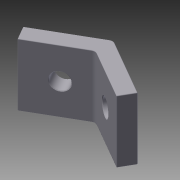
# Autodesk Inventor part: drive_frame_bracket
Saved by Autodesk Inventor 2012 (Build 160160000, 160)
## iProperties
Created: 2012-10-26
Part Number: drive_frame_bracket
Material: Aluminum-6061
Document SubType Name: Modeling
Designer: agmlego
Mass: 115.378 g
Surface Area: 72.2331 cm^2
Volume: 42.5748 cm^3
Density: 2.71 g/cm^3
Author: agmlego
Autodesk Inventor part; units mm, degrees
ref_plane "YZ Plane" through (0, 0, 0) normal (1, 0, 0) x (0, 1, 0)
ref_plane "XZ Plane" through (0, 0, 0) normal (0, 1, 0) x (-1, 0, 0)
ref_plane "XY Plane" through (0, 0, 0) normal (0, 0, 1) x (1, 0, 0)
sketch "Sketch1" plane through (0, 0, 0) normal (0, 0, 1) x (1, 0, 0)
  line L0 (-0.0175, -6.5307) -> (-20.2143, -18.1913)
  line L1 (-23.3893, -12.6921) -> (-0.0175, 0.8017)
  line L2 (-0.0175, 0.8017) -> (23.3544, -12.6921)
  line L3 (20.1794, -18.1913) -> (-0.0175, -6.5307)
  line L4 (-0.0175, 0.8017) -> (-0.0175, -6.5307) construction
  line L5 (-20.2143, -18.1913) -> (-23.3893, -12.6921)
  line L6 (20.1794, -18.1913) -> (23.3544, -12.6921)
  dimension "d4" = 120
  dimension "d5" = 6.35
  dimension "d6" = 26.9875
  constraints: 14 end point, 2 equal length, 2 parallel, 2 perpendicular
  measures "d4" angle of L2 L1
  measures "d5" distance between parallel lines of L0 L1
  measures "d6" distance from line of L1.end L5
extrude "Extrusion1" add sketch "Sketch1" along normal blind 25.4
hole "Hole1" at (9.1809, -11.8413, 12.7) direction (0.5, 0.8660254, 0) diameter 6.756 end through all clearance for "Flat Head Machine Screw (82)" size "1/4" standard "Ansi Unified Screw Threads"
hole "Hole2" at (-9.2158, -11.8413, 12.7) direction (-0.5, 0.8660254, 0) diameter 6.756 end through all clearance for "Flat Head Machine Screw (82)" size "1/4" standard "Ansi Unified Screw Threads"
fillet "Fillet1" radius 2 2 edges at (-0.0175, -6.5307, 12.7) (-0.0175, 0.8017, 12.7)
fillet "Fillet2" radius 0.25 20 edges at (-23.3893, -12.6921, 12.7) (-20.2143, -18.1913, 12.7) (20.1794, -18.1913, 12.7) (23.3544, -12.6921, 12.7) (-0.0175, 0.4923, 25.4) (-12.2034, -6.2339, 25.4) (12.1685, -6.2339, 25.4) (-0.0175, -6.8401, 25.4) (-10.6159, -12.6497, 25.4) (10.581, -12.6497, 25.4) (-21.8018, -15.4417, 25.4) (21.7669, -15.4417, 25.4) (-21.8018, -15.4417, 0) (-0.0175, 0.4923, 0) (12.1685, -6.2339, 0) (-12.2034, -6.2339, 0) (-0.0175, -6.8401, 0) (10.581, -12.6497, 0) (-10.6159, -12.6497, 0) (21.7669, -15.4417, 0)
chamfer "Chamfer1" distance 0.25 angle 45 4 edges at (-9.2158, -11.8413, 16.078) (9.1809, -11.8413, 16.078) (-12.3908, -6.3421, 16.078) (12.3559, -6.3421, 16.078)
body "Solid1"
